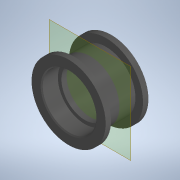
# Autodesk Inventor part: idler pulley
Saved by Autodesk Inventor 2020.3 (Build 243373000, 373)
## iProperties
Created: 2016-04-12
Part Number: idler pulley
Material: Generic
Document SubType Name: Modeling
Designer: Ben
Density: 1 g/cm^3
Appearance: Default
Author: Ben
Autodesk Inventor part; units mm, degrees
ref_plane "YZ Plane" through (0, 0, 0) normal (1, 0, 0) x (0, 1, 0)
ref_plane "XZ Plane" through (0, 0, 0) normal (0, 1, 0) x (-1, 0, 0)
ref_plane "XY Plane" through (0, 0, 0) normal (0, 0, 1) x (1, 0, 0)
sketch "Sketch1" plane through (0, 0, 0) normal (1, 0, 0) x (0, 1, 0)
  line L0 (7.987, -6.35) -> (11, -6.35)
  line L1 (11, -6.35) -> (11, -4.75)
  line L2 (11, -4.75) -> (8.75, -4.75)
  line L3 (8.75, -4.75) -> (8.75, 4.75)
  line L4 (8.75, 4.75) -> (11, 4.75)
  line L5 (11, 4.75) -> (11, 6.35)
  line L6 (11, 6.35) -> (7.987, 6.35)
  line L7 (7.987, 6.35) -> (7.987, 1.55)
  line L8 (7.987, 1.55) -> (6.945, 1.55)
  line L9 (6.945, 1.55) -> (6.945, -1.55)
  line L10 (6.945, -1.55) -> (7.987, -1.55)
  line L11 (7.987, -1.55) -> (7.987, -6.35)
  line L12 (0, 0) -> (0, 23.3621) construction
  line L13 (6.945, 0) -> (8.75, 0) construction
  dimension "d0" = 9.5
  dimension "d1" = 15.974
  dimension "d2" = 13.89
  dimension "d3" = 3.1
  dimension "d4" = 12.7
  dimension "d5" = 17.5
  dimension "d6" = 22
  constraints: 28 end point, 10 parallel, 3 collinear, 2 midpoint, 2 perpendicular, 1 horizontal, 1 point on line, 1 other
  measures "d0" distance between parallel lines of L2 L4
  measures "d1" diameter of L11 L12
  measures "d2" diameter of L9 L12
  measures "d3" distance between parallel lines of L10 L8
  measures "d4" distance between parallel lines of L0 L6
  measures "d5" diameter of L3 L12
  measures "d6" diameter of L5 L12
revolve "Revolution1" add sketch "Sketch1" angle 360 about axis through (0, 0, 0) along (0, 0, 1)
chamfer "Chamfer1" distance 0.3 angle 45 2 edges at (0, -7.987, 6.35) (0, -7.987, -6.35)
ref_plane "Work Plane1" through (0, 0, 0) normal (0, 0, -1) x (-1, 0, 0)
body "Solid1"
